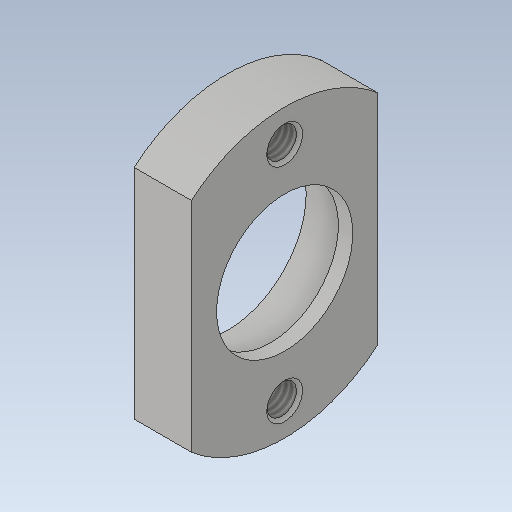
# Autodesk Inventor part: SBGTN6900VV_h
Saved by Autodesk Inventor 2020.2 (Build 242310000, 310)
## iProperties
Created: 2022-11-14
Part Number: SBGTN6900VV_h
Material: Generic
Catalog Web Link: www.cadenas.de
Description: BGTNB, BGTN, SBGTN_housing-Bearings with Housings - Space Saving, Small Flange - Non-Retained
Vendor: MISUMI
Document SubType Name: Modeling
Designer: psAdmin
Manufacturer: MISUMI
Mass: 4.62204 g
Surface Area: 29.706 cm^2
Volume: 4.62204 cm^3
Density: 1 g/cm^3
Appearance: PSOLRGB-175-175-175
Category: PARTsolutions
Company: MISUMI
PSOL_IDENT_0: {$CADENAS_DATA/23d-libs/misumi/metric/12_bearing_holders/bgtnb/housing_bgtnb.prj},201 {VTYP=3D},{NB=
PSOL_IDENT_1: SBGTN6900VV_h},{LINA=SBGTN6900VV},{NN=BGTNB, BGTN, SBGTN_housing},{DATE=25.04.2017 02:57:07},{GEOMDA
PSOL_IDENT_2: TE=10.07.2015 02:20:10},{VERSION=},{LINEID=90},{WBVAR=MATB,ST,SEAL,ALT1},{WBNUMERIC=}  {NB=SBGTN6900
PSOL_IDENT_3: VV_h},{LINA=SBGTN6900VV},{KT=DUMMY},{PN=SBGTN6900VV},{TYPE=SBGTN},{MATB=SS},{MATBALG= 'S' , 'Steel'
PSOL_IDENT_4: , 'SS' , 'Stainless Steel' },{ST=-},{STALG= '-' , '-' },{BN=6900},{SEAL=VV},{SEALALG= 'ZZ' , 'Double
PSOL_IDENT_5: Shielded' , 'VV' , 'Non-Contact Sealed Rubber Seal' , 'DD' , 'Contact Sealed Rubber Seal' },{DD=10}
PSOL_IDENT_6: ,{D=22},{B=6},{H=40},{W=26},{T=8},{DDHH=19},{A=31},{F=0},{M=M5},{ALT1=},{M3D=5}
NB: SBGTN6900VV_h
NN: BGTNB, BGTN, SBGTN_housing
NT: Bearings with Housings - Space Saving, Small Flange - Non-Retained
NBSYN: $PN._h
LINA: SBGTN6900VV
CATALOG: Misumi
PN: SBGTN6900VV
MATB: Stainless Steel
ST: -
BN: 6900
SEAL: Non-Contact Sealed Rubber Seal
DD: 10
D: 22
B: 6
H: 40
W: 26
T: 8
DDHH: 19
A: 31
F: 0
M: M5
ALT1: Bearing and Retaining Ring Assembled
SUPPLIER: MISUMI
ARTICLENO: SBGTN6900VV_h
BOMINFO: SBGTN6900VV
CREATOR: CADENAS GmbH
Title: SBGTN6900VV
Author: Cadenas PARTsolutions
Comments: Bearings with Housings - Space Saving, Small Flange - Non-Retained
Autodesk Inventor part; units mm, degrees
sketch "Sketch_1" plane through (0, 0, 0) normal (1, 0, 0) x (0, 0, -1)
  line L0 (-13, 15.1987) -> (-13, -15.1987)
  arc A0 (-13, -15.1987) -> (13, -15.1987) centre (0, 0) ccw
  line L1 (13, -15.1987) -> (13, 15.1987)
  arc A1 (13, 15.1987) -> (-13, 15.1987) centre (0, 0) ccw
  constraints: 4 end point, 4 point on circle, 2 centre point
extrude "Extrusion1" add sketch "Sketch_1" along normal mid plane 8
sketch "Sketch2" plane through (-4, 0, 0) normal (-1, 0, 0) x (0, 0, 1)
  point P0 (0, 0)
hole "Hole1" at (-4, 0, 0) direction (1, 0, 0) diameter 19 depth 8 counterbore diameter 22 counterbore depth 6
sketch "Sketch_11" plane through (0, 0, 0) normal (0, 0, 1) x (1, 0, 0)
  line L0 (4, -15.5) -> (-4, -15.5)
  line L1 (-4, -15.5) -> (-4, -13)
  line L2 (-4, -13) -> (-3.567, -13.433)
  line L3 (-3.567, -13.433) -> (3.567, -13.433)
  line L4 (3.567, -13.433) -> (4, -13)
  line L5 (4, -13) -> (4, -15.5)
  line L6 (4, -15.5) -> (-4, -15.5)
  constraints: 14 end point
revolve "Revolution1" cut sketch "Sketch_11" angle 360 about axis through (4, -15.5, 0) along (1, 0, 0)
thread "Thread1" size "M5x0.8" class "6H" standard "ISO Metric profile" full length
sketch "Sketch_9" plane through (0, 0, 0) normal (0, 0, 1) x (1, 0, 0)
  line L0 (4, 15.5) -> (-4, 15.5)
  line L1 (-4, 15.5) -> (-4, 18)
  line L2 (-4, 18) -> (-3.567, 17.567)
  line L3 (-3.567, 17.567) -> (3.567, 17.567)
  line L4 (3.567, 17.567) -> (4, 18)
  line L5 (4, 18) -> (4, 15.5)
  line L6 (4, 15.5) -> (-4, 15.5)
  constraints: 14 end point
revolve "Revolution2" cut sketch "Sketch_9" angle 360 about axis through (4, 15.5, 0) along (1, 0, 0)
thread "Thread2" size "M5x0.8" class "6H" standard "ISO Metric profile" full length
ref_plane "housing_to_dummy_XY" through (0, 0, 0) normal (0, 0, 1) x (1, 0, 0)
ref_plane "housing_to_dummy_YZ" through (0, 0, 0) normal (1, 0, 0) x (0, 1, 0)
ref_plane "housing_to_dummy_ZX" through (0, 0, 0) normal (0, 1, 0) x (0, 0, 1)
ref_plane "to_bearings_XY" through (-4, 0, 0) normal (-1, 0, 0) x (0, 0, -1)
ref_plane "to_bearings_YZ" through (-4, 0, 0) normal (0, 0, -1) x (0, -1, 0)
ref_plane "to_bearings_ZX" through (-4, 0, 0) normal (0, -1, 0) x (-1, 0, 0)
body "Solid1"
